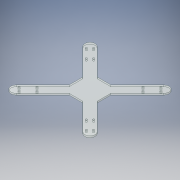
# Autodesk Inventor part: drone frame
Saved by Autodesk Inventor 2019.4 (Build 234330000, 330)
## iProperties
Created: 2019-06-03
Part Number: drone frame
Material: Generic
Document SubType Name: Modeling
Designer: abdel
Density: 1 g/cm^3
Appearance: Clear
Author: abdel
Autodesk Inventor part; units mm, degrees
ref_plane "YZ Plane" through (0, 0, 0) normal (1, 0, 0) x (0, 1, 0)
ref_plane "XZ Plane" through (0, 0, 0) normal (0, 1, 0) x (-1, 0, 0)
ref_plane "XY Plane" through (0, 0, 0) normal (0, 0, 1) x (1, 0, 0)
sketch "Sketch1" plane through (0, 0, 0) normal (0, 1, 0) x (-1, 0, 0)
  line L0 (-16.1896, 16.1896) -> (10.7512, 43.1304)
  line L1 (-295.5896, -16.1896) -> (-322.5304, 10.7512)
  line L2 (16.1896, -263.2104) -> (43.1304, -290.1512)
  line L3 (-43.1304, -268.6488) -> (10.7512, -322.5304)
  line L4 (-10.7512, -236.2696) -> (16.1896, -263.2104)
  line L5 (-295.5896, -263.2104) -> (-268.6488, -236.2696)
  line L6 (-290.1512, -322.5304) -> (-236.2696, -268.6488)
  line L7 (-322.5304, -290.1512) -> (-295.5896, -263.2104)
  arc A0 (-290.1512, 43.1304) -> (-322.5304, 10.7512) centre (-306.3408, 26.9408) ccw
  arc A1 (-322.5304, -290.1512) -> (-290.1512, -322.5304) centre (-306.3408, -306.3408) ccw
  arc A2 (10.7512, -322.5304) -> (43.1304, -290.1512) centre (26.9408, -306.3408) ccw
  arc A3 (43.1304, 10.7512) -> (10.7512, 43.1304) centre (26.9408, 26.9408) ccw
  line L8 (-329.2363, 49.8363) -> (49.8363, 49.8363)
  line L9 (49.8363, -329.2363) -> (49.8363, 49.8363)
  line L10 (49.8363, -329.2363) -> (-329.2363, -329.2363)
  line L11 (-329.2363, 49.8363) -> (-329.2363, -329.2363)
  line L12 (-10.7512, -236.2696) -> (-76.2, -170.8208)
  line L13 (-170.8208, -76.2) -> (-290.1512, 43.1304)
  line L14 (-43.1304, -268.6488) -> (-108.5792, -203.2)
  line L15 (-203.2, -108.5792) -> (-295.5896, -16.1896)
  line L16 (-236.2696, -268.6488) -> (-170.8208, -203.2)
  line L17 (-76.2, -108.5792) -> (43.1304, 10.7512)
  line L18 (-268.6488, -236.2696) -> (-203.2, -170.8208)
  line L19 (-108.5792, -76.2) -> (-16.1896, 16.1896)
  line L20 (-108.5792, -76.2) -> (-170.8208, -76.2)
  line L21 (-203.2, -108.5792) -> (-203.2, -170.8208)
  line L22 (-170.8208, -203.2) -> (-108.5792, -203.2)
  line L23 (-76.2, -170.8208) -> (-76.2, -108.5792)
  circle A4 centre (2254.858, -433.3281) radius 4.2386
  circle A5 centre (2254.858, -433.3281) radius 14.0056
  line L24 (2254.858, -433.3281) -> (2238.6684, -449.5177)
  line L25 (2254.858, -433.3281) -> (2271.0476, -417.1385)
  line L26 (2238.6684, -449.5177) -> (2211.7277, -422.5769)
  line L27 (2271.0476, -417.1385) -> (2297.9884, -444.0792)
  line L28 (2211.7277, -422.5769) -> (2265.6092, -476.4584)
  line L29 (2265.6092, -476.4584) -> (2297.9884, -444.0792)
  line L30 (2297.9884, -444.0792) -> (2244.1069, -390.1977)
  line L31 (2244.1069, -390.1977) -> (2211.7277, -422.5769)
  line L32 (-29.66, -282.1192) -> (-43.1304, -268.6488)
  line L33 (-43.1304, -268.6488) -> (-29.66, -282.1192)
  line L34 (2.7192, -249.74) -> (-10.7512, -236.2696)
  line L35 (-10.7512, -236.2696) -> (-43.1304, -268.6488)
  line L36 (-43.1304, -268.6488) -> (-29.66, -282.1192)
  line L37 (-29.66, -282.1192) -> (2.7192, -249.74)
  line L38 (-43.1304, -268.6488) -> (-36.3952, -275.384)
  circle A6 centre (-28.2995, -267.2883) radius 4.445
  circle A7 centre (-12.1081, -251.0969) radius 4.445
  line L39 (10.7512, -322.5304) -> (43.1304, -290.1512)
  circle A8 centre (28.3031, -291.5081) radius 4.445
  line L40 (43.1304, -290.1512) -> (29.66, -276.6808)
  line L41 (29.66, -276.6808) -> (-2.7192, -309.06)
  line L42 (29.66, -276.6808) -> (-2.7192, -309.06)
  circle A9 centre (12.1117, -307.6995) radius 4.445
  line L43 (10.7512, -322.5304) -> (-2.7192, -309.06)
  line L44 (-2.7192, -309.06) -> (10.7512, -322.5304)
  line L45 (-2.7192, -309.06) -> (4.016, -315.7952)
  line L46 (-2.7192, -309.06) -> (10.7512, -322.5304)
  line L47 (-76.2, -170.8208) -> (-114.6919, -170.8208)
  circle A10 centre (-279.4, 0) radius 4.2386
  circle A11 centre (-279.4, 0) radius 14.0056
  line L48 (-322.5304, 10.7512) -> (-268.6488, -43.1304)
  line L49 (-236.2696, -10.7512) -> (-290.1512, 43.1304)
  line L50 (-268.6488, -43.1304) -> (-236.2696, -10.7512)
  line L51 (-263.2104, 16.1896) -> (-236.2696, -10.7512)
  line L52 (-279.4, 0) -> (-295.5896, -16.1896)
  line L53 (-279.4, 0) -> (-263.2104, 16.1896)
  circle A12 centre (-291.5081, 28.3031) radius 4.445
  line L54 (-309.06, -2.7192) -> (-276.6808, 29.66)
  line L55 (-276.6808, 29.66) -> (-290.1512, 43.1304)
  line L56 (-290.1512, 43.1304) -> (-322.5304, 10.7512)
  line L57 (-290.1512, 43.1304) -> (-322.5304, 10.7512)
  circle A13 centre (-307.6995, 12.1117) radius 4.445
  line L58 (-295.5896, -16.1896) -> (-322.5304, 10.7512)
  line L59 (-309.06, -2.7192) -> (-322.5304, 10.7512)
  line L60 (-322.5304, 10.7512) -> (-309.06, -2.7192)
  line L61 (-322.5304, 10.7512) -> (-309.06, -2.7192)
  line L62 (-322.5304, 10.7512) -> (-315.7952, 4.016)
  circle A14 centre (-251.0969, -12.1081) radius 4.445
  line L63 (-249.74, 2.7192) -> (-282.1192, -29.66)
  line L64 (-249.74, 2.7192) -> (-282.1192, -29.66)
  line L65 (-282.1192, -29.66) -> (-275.384, -36.3952)
  circle A15 centre (-267.2883, -28.2995) radius 4.445
  line L66 (-268.6488, -43.1304) -> (-236.2696, -10.7512)
  line L67 (-268.6488, -43.1304) -> (-282.1192, -29.66)
  line L68 (-282.1192, -29.66) -> (-268.6488, -43.1304)
  line L69 (-282.1192, -29.66) -> (-268.6488, -43.1304)
  line L70 (-236.2696, -10.7512) -> (-249.74, 2.7192)
  circle A16 centre (0, 0) radius 4.2386
  circle A17 centre (0, 0) radius 14.0056
  line L71 (-10.7512, -43.1304) -> (43.1304, 10.7512)
  line L72 (10.7512, 43.1304) -> (-43.1304, -10.7512)
  line L73 (43.1304, 10.7512) -> (10.7512, 43.1304)
  line L74 (-16.1896, 16.1896) -> (10.7512, 43.1304)
  line L75 (0, 0) -> (16.1896, -16.1896)
  line L76 (0, 0) -> (-16.1896, 16.1896)
  circle A18 centre (-28.3031, -12.1081) radius 4.445
  line L77 (2.7192, -29.66) -> (-29.66, 2.7192)
  line L78 (-29.66, 2.7192) -> (-43.1304, -10.7512)
  line L79 (-43.1304, -10.7512) -> (-10.7512, -43.1304)
  line L80 (-43.1304, -10.7512) -> (-10.7512, -43.1304)
  circle A19 centre (-12.1117, -28.2995) radius 4.445
  line L81 (16.1896, -16.1896) -> (-10.7512, -43.1304)
  line L82 (2.7192, -29.66) -> (-10.7512, -43.1304)
  line L83 (-10.7512, -43.1304) -> (2.7192, -29.66)
  line L84 (-10.7512, -43.1304) -> (2.7192, -29.66)
  line L85 (-10.7512, -43.1304) -> (-4.016, -36.3952)
  circle A20 centre (12.1081, 28.3031) radius 4.445
  line L86 (-2.7192, 29.66) -> (29.66, -2.7192)
  line L87 (-2.7192, 29.66) -> (29.66, -2.7192)
  line L88 (29.66, -2.7192) -> (36.3952, 4.016)
  circle A21 centre (28.2995, 12.1117) radius 4.445
  line L89 (43.1304, 10.7512) -> (10.7512, 43.1304)
  line L90 (43.1304, 10.7512) -> (29.66, -2.7192)
  line L91 (29.66, -2.7192) -> (43.1304, 10.7512)
  line L92 (29.66, -2.7192) -> (43.1304, 10.7512)
  line L93 (10.7512, 43.1304) -> (-2.7192, 29.66)
  circle A22 centre (-291.5117, -307.6995) radius 4.445
  circle A23 centre (-307.7031, -291.5081) radius 4.445
  line L94 (-309.06, -276.6808) -> (-322.5304, -290.1512)
  line L95 (-276.6808, -309.06) -> (-290.1512, -322.5304)
  line L96 (-290.1512, -322.5304) -> (-276.6808, -309.06)
  line L97 (-290.1512, -322.5304) -> (-276.6808, -309.06)
  line L98 (-263.2104, -295.5896) -> (-290.1512, -322.5304)
  line L99 (-268.6488, -236.2696) -> (-322.5304, -290.1512)
  line L100 (-290.1512, -322.5304) -> (-236.2696, -268.6488)
  line L101 (-290.1512, -322.5304) -> (-283.416, -315.7952)
  line L102 (-268.6488, -236.2696) -> (-282.1192, -249.74)
  circle A24 centre (-267.2919, -251.0969) radius 4.445
  line L103 (-295.5896, -263.2104) -> (-268.6488, -236.2696)
  circle A25 centre (-251.1005, -267.2883) radius 4.445
  line L104 (-249.74, -282.1192) -> (-243.0048, -275.384)
  line L105 (-249.74, -282.1192) -> (-236.2696, -268.6488)
  line L106 (-249.74, -282.1192) -> (-236.2696, -268.6488)
  line L107 (-236.2696, -268.6488) -> (-249.74, -282.1192)
  line L108 (-290.1512, -322.5304) -> (-322.5304, -290.1512)
  point P0 (-279.4, 0)
  point P1 (-279.4, -279.4)
  dimension "d68" = 379.0727
  dimension "d69" = 379.0727
  dimension "d70" = 379.0727
  dimension "d77" = 45.7911
  dimension "d78" = 8.4772
  dimension "d79" = 28.0111
  dimension "d80" = 22.8956
  dimension "d81" = 22.8956
  dimension "d82" = 38.1
  dimension "d83" = 38.1
  dimension "d84" = 45.7962
  dimension "d85" = 76.2
  dimension "d86" = 45.7911
  dimension "d87" = 19.05
  dimension "d88" = 19.05
  dimension "d89" = 9.525
  dimension "d90" = 8.89
  dimension "d91" = 45.7911
  dimension "d92" = 45.7911
  dimension "d93" = 19.05
  dimension "d94" = 19.05
  dimension "d95" = 9.525
  dimension "d96" = 8.89
  dimension "d97" = 135
  dimension "d98" = 8.4772
  dimension "d99" = 28.0111
  dimension "d100" = 22.8956
  dimension "d101" = 22.8956
  dimension "d102" = 38.1
  dimension "d103" = 38.1
  dimension "d104" = 45.7911
  dimension "d105" = 76.2
  dimension "d106" = 45.7911
  dimension "d107" = 19.05
  dimension "d108" = 19.05
  dimension "d109" = 9.525
  dimension "d110" = 8.89
  dimension "d111" = 45.7911
  dimension "d112" = 45.7911
  dimension "d113" = 19.05
  dimension "d114" = 19.05
  dimension "d115" = 9.525
  dimension "d116" = 8.89
  dimension "d117" = 8.4772
  dimension "d118" = 28.0111
  dimension "d119" = 22.8956
  dimension "d120" = 22.8956
  dimension "d121" = 38.1
  dimension "d122" = 38.1
  dimension "d123" = 45.7962
  dimension "d124" = 76.2
  dimension "d125" = 45.7911
  dimension "d126" = 19.05
  dimension "d127" = 19.05
  dimension "d128" = 9.525
  dimension "d129" = 8.89
  dimension "d130" = 45.7911
  dimension "d131" = 45.7911
  dimension "d132" = 19.05
  dimension "d133" = 19.05
  dimension "d134" = 9.525
  dimension "d135" = 8.89
  dimension "d140" = 38.1
  dimension "d141" = 38.1
  constraints: 218 end point, 26 centre point, 17 parallel, 10 perpendicular, 8 midpoint, 8 point on circle, 8 tangent, 6 coincident, 4 horizontal, 2 vertical
  measures "d68" distance of L9.start L8.end
  measures "d69" distance of L8.start L10.end
  measures "d70" distance of L9.start L10.end
  measures "d77" distance between parallel lines of L4 L3
  measures "d78" diameter of A4
  measures "d79" diameter of A5
  measures "d80" distance of L24.start L24.end
  measures "d81" distance of L24.start L27.start
  measures "d82" distance of L24.end L28.start
  measures "d83" distance of L27.start L30.start
  measures "d85" distance of L30.start L30.end
  measures "d86" distance of L34.end L35.end
  measures "d87" distance of L37.end L34.end
  measures "d88" distance of L37.start L35.end
  measures "d89" distance of L35.end L38.end
  measures "d90" diameter of A6
  measures "d91" distance of L41.start L41.end
  measures "d92" distance of L42.start L42.end
  measures "d93" distance of L39.end L42.start
  measures "d94" distance of L39.start L42.end
  measures "d95" distance of L42.end L45.end
  measures "d96" diameter of A9
  measures "d97" angle of L12 L47
  measures "d98" diameter of A10
  measures "d99" diameter of A11
  measures "d100" distance of L52.start L58.start
  measures "d101" distance of L52.start L51.start
  measures "d102" distance of L58.start L58.end
  measures "d103" distance of L51.start L49.start
  measures "d104" distance of L49.end L58.end
  measures "d105" distance of L49.start L49.end
  measures "d106" distance of L57.start L57.end
  measures "d107" distance of L55.start L57.start
  measures "d108" distance of L59.start L57.end
  measures "d109" distance of L57.end L62.end
  measures "d110" diameter of A13
  measures "d111" distance of L63.start L63.end
  measures "d112" distance of L70.end L64.end
  measures "d113" distance of L70.start L70.end
  measures "d114" distance of L66.start L64.end
  measures "d115" distance of L64.end L65.end
  measures "d116" diameter of A15
  measures "d117" diameter of A16
  measures "d118" diameter of A17
  measures "d119" distance of L75.start L81.start
  measures "d120" distance of L75.start L74.start
  measures "d121" distance of L81.start L81.end
  measures "d122" distance of L74.start L72.start
  measures "d124" distance of L72.start L72.end
  measures "d125" distance of L80.start L80.end
  measures "d126" distance of L78.start L80.start
  measures "d127" distance of L82.start L80.end
  measures "d128" distance of L80.end L85.end
  measures "d129" diameter of A19
  measures "d130" distance of L86.start L86.end
  measures "d131" distance of L93.end L87.end
  measures "d132" distance of L93.start L93.end
  measures "d133" distance of L89.start L87.end
  measures "d134" distance of L87.end L88.end
  measures "d135" diameter of A21
  measures "d140" distance of L98.start L98.end
  measures "d141" distance of L103.start L103.end
extrude "Extrusion2" add sketch "Sketch1" along normal blind 7.112 contours L76 A17 L75 L17 L77 L19 | L0 L86 L17 L75 A17 L76 | L0 L73 L17 L86 | L77 L17 L79 L19 | L76 A16 L75 A17 | A17 L75 A16 L76 | A3 L73 | L79 L17 L23 L12 L35 L14 L22 L16 L6 L108 L7 L5 L18 L21 L15 L50 L13 L20 L19 | L76 L75 A16 | A16 L75 L76 | A0 L56 | A2 L39 | L13 L54 L1 L56 | L50 L15 L63 L13 | L39 L3 L41 L2 | L13 L53 A11 L52 L1 L54 | A1 L108 | L63 L15 L52 A11 L53 L13 | L4 L37 L3 L35 | L41 L3 L37 L4 L2 | L53 A10 L52 A11 | A11 L52 A10 L53 | L53 L52 A10 | A10 L52 L53
body "Solid2"
